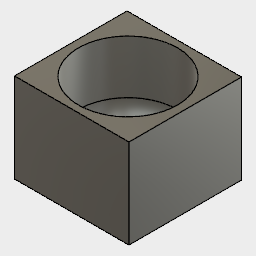
hållare till kulorna (Autodesk Fusion 360 design; units mm, degrees)
Autodesk Fusion 360 part; units mm, degrees
sketch "Sketch1" plane through (0, 0, 0) normal (0, 1, 0) x (1, 0, 0)
  line L0 (0, 0) -> (12, 0)
  line L1 (12, 0) -> (12, -12)
  line L2 (12, -12) -> (0, -12)
  line L3 (0, -12) -> (0, 0)
  dimension "d1" = 12
  dimension "d2" = 12
  measures "d1" distance of L0.start L2.end
  measures "d2" distance of L0.start L0.end
extrude "Extrude1" add sketch "Sketch1" along normal blind 9.2
sketch "Sketch9" plane through (0, 9.2, 0) normal (0, 1, 0) x (-1, 0, 0)
  line L0 (0, 12) -> (-12, 12)
  line L1 (-12, 12) -> (-12, 0)
  line L2 (-12, 0) -> (0, 0)
  line L3 (0, 0) -> (0, 12)
  circle A0 centre (-6, 6) radius 5.1
  dimension "d6" = 10.2
  measures "d6" diameter of A0
extrude "Extrude2" cut sketch "Sketch9" against normal blind 5.5 contours A0
sphere "SpherePrimitive2" cut diameter 10.2 placed x (-1, 0, 0) y (0, 0, 1) z (0, 1, 0) at (6, 3.7, 6)
extrude "Extrude3" cut 1 faces at (0, 3.0667, 8) along direction (1, 0, 0) blind 0.1
extrude "Extrude4" cut 1 faces at (12, 3.0667, 4) along direction (-1, 0, 0) blind 0.1
extrude "Extrude5" cut 1 faces at (4.0333, 3.0667, 0) along direction (0, 0, 1) blind 0.2
extrude "Extrude6" cut 1 faces at (7.9667, 3.0667, 12) along direction (0, 0, -1) blind 0.2
